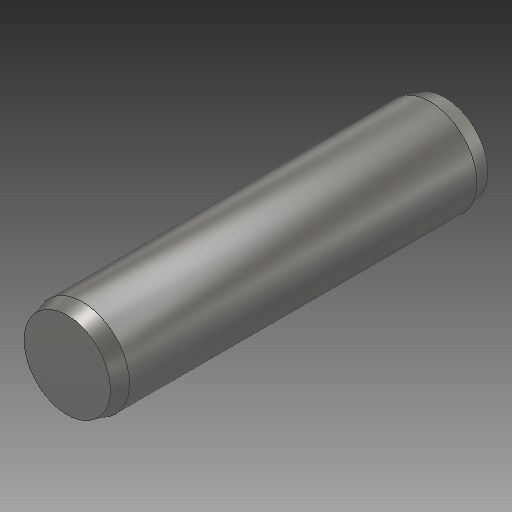
# Autodesk Inventor part: φ2.5ピン 10
Saved by Autodesk Inventor 2017.3 (Build 213256000, 256)
## iProperties
Part Number: φ2.5ピン 10
Material: ステンレス鋼
Document SubType Name: Modeling
Designer: 原知也
Density: 8 g/cm^3
Appearance: 半つや出し
Mass: 0.390082 g
Surface Area: 0.866887 cm^2
Volume: 0.0487603 cm^3
Author: 原知也
Autodesk Inventor part; units mm, degrees
ref_plane "YZ Plane" through (0, 0, 0) normal (1, 0, 0) x (0, 1, 0)
ref_plane "XZ Plane" through (0, 0, 0) normal (0, 1, 0) x (-1, 0, 0)
ref_plane "XY Plane" through (0, 0, 0) normal (0, 0, 1) x (1, 0, 0)
sketch "スケッチ2" plane through (0, 0, 0) normal (1, 0, 0) x (0, 1, 0)
  line L0 (0, 9.3427) -> (0, -26.8463) construction
  line L1 (1.25, 0) -> (-22.4246, 0) construction
  line L2 (0, 5) -> (1.1428, 5)
  line L3 (1.25, 0) -> (1.25, 4.6)
  line L4 (1.25, 4.6) -> (1.25, 5) construction
  line L5 (1.25, 4.6) -> (1.1428, 5)
  line L6 (1.1428, 5) -> (1.25, 5) construction
  line L7 (0, -5) -> (1.1428, -5)
  line L8 (1.25, 0) -> (1.25, -4.6)
  line L9 (1.25, -4.6) -> (1.25, -5) construction
  line L10 (1.25, -4.6) -> (1.1428, -5)
  line L11 (1.1428, -5) -> (1.25, -5) construction
  line L12 (0, 5) -> (0, -5)
  point P0 (0, 0)
  dimension "d0" = 1.25
  dimension "d1" = 5
  dimension "d2" = 0.4
  dimension "d3" = 15
  constraints: 26 end point, 4 symmetric about line, 3 horizontal, 3 vertical, 1 collinear, 1 point on line
  measures "d0" distance of L1.start point (0, 0)
  measures "d1" distance between parallel lines of L1 L2
  measures "d2" distance of L4.end L3.end
  measures "d3" angle of L5 L4
revolve "回転1" add sketch "スケッチ2" angle 360 about axis through (0, 0, 9.3427) along (0, 0, -1)
